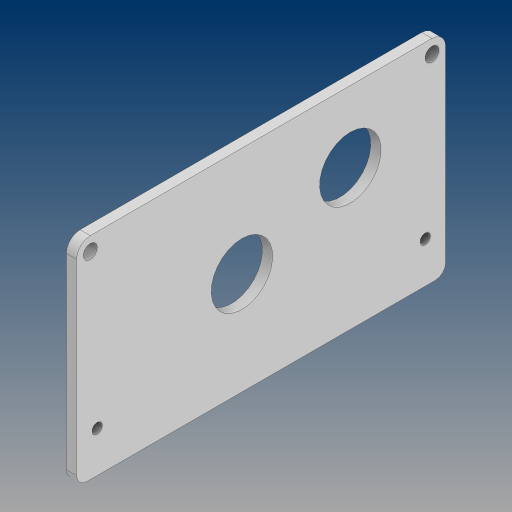
# Autodesk Inventor part: Intake Pivot Gearbox
Saved by Autodesk Inventor 2024.3 (Build 283343000, 343)
## iProperties
Created: 2024-08-01
Part Number: Intake Pivot Gearbox
Material: Generic
Document SubType Name: Modeling
Designer: Kenji
Density: 1 g/cm^3
Appearance: Default
Author: Kenji
Autodesk Inventor part; units mm, degrees
ref_plane "YZ Plane" through (0, 0, 0) normal (1, 0, 0) x (0, 1, 0)
ref_plane "XZ Plane" through (0, 0, 0) normal (0, 1, 0) x (-1, 0, 0)
ref_plane "XY Plane" through (0, 0, 0) normal (0, 0, 1) x (1, 0, 0)
sketch "Sketch1" plane through (0, 0, 0) normal (1, 0, 0) x (0, 1, 0)
  circle A0 centre (65.1002, 0) radius 14.2875
  circle A1 centre (65.1002, 0) radius 31.115 construction
  circle A2 centre (65.1002, 93.9109) radius 10.16
  circle A3 centre (47.4853, 50.3475) radius 36.83 construction
  circle A4 centre (47.4853, 50.3475) radius 22.86 construction
  circle A5 centre (65.1002, 0) radius 30.48 construction
  circle A6 centre (65.1002, 93.9109) radius 30 construction
  circle A7 centre (65.1002, 93.9109) radius 25.4 construction
  circle A8 centre (47.4853, 50.3475) radius 14.2875
  circle A9 centre (47.4853, 50.3475) radius 7.62 construction
  circle A10 centre (19.05, -34.7726) radius 2.3812
  circle A11 centre (19.05, 117.6274) radius 2.3876
  circle A12 centre (47.4853, 50.3475) radius 38.1 construction
  circle A13 centre (65.1002, 0) radius 31.75 construction
  circle A14 centre (91.7702, 120.8024) radius 6.35 construction
  circle A15 centre (91.7702, -37.9476) radius 6.35 construction
  line L0 (88.1189, -32.7523) -> (83.3566, -25.9763) construction
  line L1 (98.1202, 120.8024) -> (98.1202, -37.9476)
  circle A16 centre (91.7702, 120.8024) radius 3.2512
  circle A17 centre (91.7702, -37.9476) radius 3.2512
  line L2 (0, 127.1524) -> (0, 108.1024) construction
  line L3 (0, 108.1024) -> (28.575, 108.1024) construction
  line L4 (28.575, 108.1024) -> (28.575, 127.1524) construction
  line L5 (28.575, -25.2476) -> (0, -25.2476) construction
  line L6 (0, -25.2476) -> (0, -44.2976) construction
  line L7 (28.575, -44.2976) -> (28.575, -25.2476) construction
  line L8 (28.3112, 127.1524) -> (91.7702, 127.1524)
  line L9 (91.7702, -44.2976) -> (28.575, -44.2976)
  line L10 (0, 122.3772) -> (0, -39.5224)
  arc A18 (91.7702, -44.2976) -> (98.1202, -37.9476) centre (91.7702, -37.9476) ccw
  arc A19 (98.1202, 120.8024) -> (91.7702, 127.1524) centre (91.7702, 120.8024) ccw
  line L11 (28.838, 127.1524) -> (4.7752, 127.1524)
  line L12 (28.575, -44.2976) -> (4.7752, -44.2976)
  arc A20 (28.575, -44.2976) -> (28.575, -44.2976) centre (28.575, -39.5224) ccw
  arc A21 (4.7752, 127.1524) -> (0, 122.3772) centre (4.7752, 122.3772) ccw
  arc A22 (0, -39.5224) -> (4.7752, -44.2976) centre (4.7752, -39.5224) ccw
  circle A23 centre (47.4853, 50.3475) radius 24.13 construction
  line L13 (90.5002, 93.9109) -> (65.1002, 93.9109) construction
  line L14 (98.1202, 0) -> (96.8502, 0) construction
  line L15 (87.2987, 116.2937) -> (86.2255, 115.2117) construction
  line L16 (65.1002, 93.9109) -> (89.7457, 100.0557) construction
  circle A24 centre (89.7457, 100.0557) radius 2.75
  circle A25 centre (78.1822, 115.683) radius 2.75
  circle A26 centre (58.9554, 118.5564) radius 2.75
  circle A27 centre (43.3282, 106.9929) radius 2.75
  circle A28 centre (40.4547, 87.7661) radius 2.75
  circle A29 centre (52.0182, 72.1389) radius 2.75
  circle A30 centre (71.245, 69.2654) radius 2.75
  circle A31 centre (86.8722, 80.829) radius 2.75
  point P0 (0, 0)
  point P1 (28.575, 117.6274)
  dimension "d10" = 60
  dimension "d0" = 28.575
  dimension "d1" = 65.1002
  dimension "d2" = 62.23
  dimension "d6" = 20.32
  dimension "d7" = 73.66
  dimension "d8" = 45.72
  dimension "d9" = 60.96
  dimension "d11" = 50.8
  dimension "d17" = 28.575
  dimension "d18" = 15.24
  dimension "d20" = 4.7625
  dimension "d22" = 4.7752
  dimension "d24" = 19.05
  dimension "d28" = 63.5
  dimension "d31" = 12.7
  dimension "d32" = 12.7
  dimension "d35" = 6.5024
  dimension "d36" = 6.5024
  dimension "d37" = 19.05
  dimension "d38" = 9.525
  dimension "d39" = 9.525
  dimension "d40" = 9.525
  dimension "d43" = 4.7752
  dimension "d45" = 4.7752
  dimension "d46" = 4.7752
  dimension "d47" = 1.27
  dimension "d48" = 117.6274
  dimension "d49" = 152.4
  dimension "d52" = 1.27
  dimension "d55" = 1.27
  dimension "d56" = 1.524
  dimension "d57" = 14
  dimension "d58" = 5.5
  dimension "d61" = 360
  constraints: 34 end point, 31 centre point, 20 point on circle, 15 coincident, 14 point on line, 13 tangent, 7 horizontal, 5 vertical alignment, 2 collinear, 2 horizontal alignment, 2 parallel, 2 perpendicular, 1 concentric, 1 midpoint, 1 vertical, 20 other
  measures "d0" diameter of A0
  measures "d1" distance of point (0, 0) A0.centre
  measures "d2" diameter of A1
  measures "d6" diameter of A2
  measures "d7" diameter of A3
  measures "d8" diameter of A4
  measures "d9" diameter of A5
  measures "d11" diameter of A7
  measures "d17" diameter of A8
  measures "d18" diameter of A9
  measures "d20" diameter of A10
  measures "d22" diameter of A11
  measures "d24" horizontal distance of point (0, 0) A10.centre
  measures "d28" diameter of A13
  measures "d31" diameter of A14
  measures "d32" diameter of A15
  measures "d35" diameter of A16
  measures "d36" diameter of A17
  measures "d37" distance of L2.end L2.start
  measures "d38" distance from line of L3 A11.centre
  measures "d39" distance of A11.centre point (28.575, 117.627)
  measures "d40" distance from line of L5 A10.centre
  measures "d43" radius of A20
  measures "d45" radius of A21
  measures "d46" radius of A22
  measures "d47" radial gap between concentric circles of A3 A12
  measures "d48" vertical distance of A11.centre point (0, 0)
  measures "d49" distance of A10.centre A11.centre
  measures "d52" radial gap between concentric circles of A4 A23
  measures "d55" distance of L14.start L14.end
  measures "d56" distance of L15.start L15.end
  measures "d57" angle of L13 L16
  measures "d58" diameter of A24
extrude "Extrusion1" add sketch "Sketch1" along normal blind 4.7625 contours A2 | A20 | L1 A18 L9 L12 A22 L10 A21 L11 L8 A19 | A24 | A25 | A26 | A27 | A28 | A29 | A30 | A31
body "Solid1"
